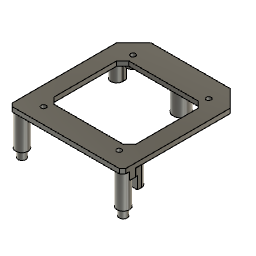
podstawka_bez_karoserii v3 (Autodesk Fusion 360 design; units mm, degrees)
Autodesk Fusion 360 part; units mm, degrees
note: some values were not read from the file. Set by a fixed rule: which face or edge a step refers to.
sketch "main" plane through (0, 0, 0) normal (0, 0, 1) x (1, 0, 0)
  circle A0 centre (50, 25) radius 4.065
  circle A1 centre (115.62, 25) radius 4.065
  circle A2 centre (50, 25) radius 2.6
  circle A3 centre (115.62, 25) radius 2.6
  line L0 (50, 29.065) -> (115.62, 29.065)
  line L1 (115.62, 29.065) -> (115.62, 90.235)
  line L2 (115.62, 90.235) -> (50, 90.235)
  line L3 (50, 90.235) -> (50, 27.6)
  line L4 (50, 29.065) -> (35.31, 29.065)
  line L5 (35.31, 29.065) -> (35.31, 90.235)
  line L6 (35.31, 90.235) -> (50, 90.235)
  line L7 (50, 90.235) -> (50, 29.065)
  line L8 (115.62, 29.065) -> (130.31, 29.065)
  line L9 (130.31, 29.065) -> (130.31, 90.235)
  line L10 (130.31, 90.235) -> (115.62, 90.235)
  line L11 (115.62, 90.235) -> (115.62, 29.065)
  line L12 (115.62, 59.65) -> (50, 59.65)
  line L13 (50, 59.65) -> (50, 90.235)
  line L14 (50, 90.235) -> (115.62, 90.235)
  line L15 (115.62, 90.235) -> (115.62, 59.65)
  line L16 (115.62, 59.65) -> (50, 90.235) construction
  line L17 (50, 59.65) -> (115.62, 90.235) construction
  line L18 (82.81, 74.9425) -> (82.81, 112.2058)
  circle A4 centre (82.81, 95.48) radius 5.245
  line L19 (82.81, 95.48) -> (88.055, 95.48)
  line L20 (82.81, 95.48) -> (77.565, 95.48)
  line L21 (77.565, 95.48) -> (77.565, 90.235)
  line L22 (88.055, 95.48) -> (88.055, 90.235)
  line L23 (50, 25) -> (54.065, 25)
  line L24 (50, 25) -> (45.935, 25)
  line L25 (54.065, 25) -> (54.065, 29.065)
  line L26 (45.935, 25) -> (45.935, 29.065)
  line L27 (115.62, 25) -> (115.62, 29.065)
  line L28 (115.62, 25) -> (119.685, 25)
  line L29 (119.685, 25) -> (119.685, 29.065)
  line L30 (111.555, 25) -> (111.555, 29.065)
  line L31 (115.62, 29.065) -> (100.93, 29.065)
  circle A5 centre (82.81, 95.48) radius 3
  line L32 (115.62, 90.235) -> (50, 29.065)
  circle A6 centre (115.62, 32.915) radius 3.85
  line L33 (115.62, 32.915) -> (119.47, 32.915)
  line L34 (115.62, 32.915) -> (111.77, 32.915)
  line L35 (119.47, 32.915) -> (119.47, 29.065)
  line L36 (111.77, 32.915) -> (111.77, 29.065)
  line L37 (115.62, 29.065) -> (50, 90.235)
  line L38 (53.85, 32.915) -> (53.85, 29.065)
  circle A7 centre (50, 32.915) radius 3.85
  line L39 (46.15, 32.915) -> (46.15, 29.065)
  line L40 (46.15, 86.385) -> (46.15, 90.235)
  circle A8 centre (50, 86.385) radius 3.85
  line L41 (53.85, 86.385) -> (53.85, 90.235)
  line L42 (111.77, 29.065) -> (119.47, 29.065)
  line L43 (119.47, 29.065) -> (119.47, 30.065)
  line L44 (119.47, 30.065) -> (111.77, 30.065)
  line L45 (111.77, 30.065) -> (111.77, 29.065)
  line L46 (46.15, 90.235) -> (53.85, 90.235)
  line L47 (53.85, 90.235) -> (53.85, 89.235)
  line L48 (53.85, 89.235) -> (46.15, 89.235)
  line L49 (46.15, 89.235) -> (46.15, 90.235)
  line L50 (50, 90.235) -> (82.81, 90.235)
  line L51 (82.81, 90.235) -> (82.81, 95.48)
  line L52 (82.81, 95.48) -> (50, 95.48)
  line L53 (50, 95.48) -> (50, 90.235)
  line L54 (130.31, 90.235) -> (82.81, 90.235)
  line L55 (82.81, 90.235) -> (82.81, 95.48)
  line L56 (50, 29.065) -> (115.62, 29.065)
  line L57 (115.62, 29.065) -> (115.62, 25)
  line L58 (115.62, 25) -> (50, 25)
  line L59 (50, 25) -> (50, 29.065)
  line L60 (45.935, 29.065) -> (119.685, 29.065)
  line L61 (119.685, 29.065) -> (119.685, 20.5)
  line L62 (119.685, 20.5) -> (45.935, 20.5)
  line L63 (45.935, 20.5) -> (45.935, 29.065)
  line L64 (88.055, 95.48) -> (115.62, 95.48)
  line L65 (115.62, 95.48) -> (115.62, 90.235)
  line L66 (115.62, 90.235) -> (88.055, 90.235)
  line L67 (88.055, 90.235) -> (88.055, 95.48)
  line L68 (50, 90.235) -> (115.62, 90.235)
  line L69 (115.62, 90.235) -> (115.62, 101.2915)
  line L70 (115.62, 101.2915) -> (50, 101.2915)
  line L71 (50, 101.2915) -> (50, 90.235)
  line L72 (46.15, 29.065) -> (46.15, 90.235)
  line L73 (119.685, 29.065) -> (119.685, 90.235)
  line L74 (119.685, 90.235) -> (115.62, 90.235)
  line L75 (115.62, 90.235) -> (115.62, 101.2915)
  line L76 (115.62, 101.2915) -> (119.685, 101.2915)
  line L77 (119.685, 101.2915) -> (119.685, 90.235)
  line L78 (46.15, 90.235) -> (50, 90.235)
  line L79 (50, 90.235) -> (50, 101.2915)
  line L80 (50, 101.2915) -> (46.15, 101.2915)
  line L81 (46.15, 101.2915) -> (46.15, 90.235)
  line L82 (82.81, 74.9425) -> (82.81, 57.8563)
  line L83 (46.15, 59.65) -> (115.62, 59.65)
  line L84 (90.31, 65.3563) -> (75.31, 65.3563)
  line L85 (75.31, 65.3563) -> (75.31, 50.3563)
  line L86 (75.31, 50.3563) -> (90.31, 50.3563)
  line L87 (90.31, 50.3563) -> (90.31, 65.3563)
  line L88 (90.31, 65.3563) -> (75.31, 50.3563) construction
  line L89 (75.31, 65.3563) -> (90.31, 50.3563) construction
  point P0 (82.81, 74.9425)
  point P1 (50, 59.65)
  point P2 (115.62, 59.65)
  point P3 (46.15, 59.65)
  point P4 (46.15, 59.65)
  point P5 (115.62, 59.65)
  point P6 (82.81, 74.9425)
  point P7 (82.81, 65.601)
  point P8 (82.81, 74.9425)
  point P9 (82.81, 57.8563)
  point P10 (82.81, 57.8563)
  dimension "d1" = 8.13
  dimension "d2" = 8.13
  dimension "d3" = 65.62
  dimension "d4" = 5.2
  dimension "d5" = 5.2
  dimension "d6" = 65.62
  dimension "d7" = 61.17
  dimension "d8" = 14.69
  dimension "d9" = 14.69
  dimension "d10" = 10.49
  dimension "d14" = 6
  dimension "d35" = 7.7
  dimension "d36" = 3.85
  dimension "d41" = 1
  dimension "d42" = 1
  dimension "d54" = 73.75
  dimension "d55" = 61.17
  dimension "d154" = 15
  dimension "d155" = 15
  constraint concentric A0 A2
  constraint concentric A1 A3
  constraint horizontal L0
  constraint vertical L1
  constraint horizontal L2
  constraint vertical L3
  constraint coincident A0 L0.start
  constraint coincident A2 L3.end
  constraint coincident L0.start L3
  constraint horizontal L4
  constraint vertical L5
  constraint horizontal L6
  constraint vertical L7
  constraint coincident L2.end L3.start
  constraint horizontal L8
  constraint vertical L9
  constraint horizontal L10
  constraint vertical L11
  constraint horizontal L12
  constraint perpendicular L12 L13
  constraint parallel L12 L14
  constraint parallel L13 L15
  constraint coincident L16 P8
  constraint coincident L17 P8
  constraint coincident L1.end L2.start
  constraint coincident P8 P6
  constraint vertical L18
  constraint coincident A4.centre L19.start
  constraint coincident A4 L19.end
  constraint perpendicular L18 L19
  constraint coincident A4 L20.end
  constraint perpendicular L18 L20
  constraint coincident L2 L21.end
  constraint tangent A4 L21
  constraint coincident L2 L22.end
  constraint tangent A4 L22
  constraint coincident A0.centre A2.centre
  constraint coincident A0 L23.end
  constraint perpendicular L3 L23
  constraint coincident A0 L24.end
  constraint parallel L23 L24
  constraint coincident L0 L25.end
  constraint tangent A0 L25
  constraint coincident L4 L26.end
  constraint tangent A0 L26
  constraint coincident A1.centre A3.centre
  constraint perpendicular L0 L27
  constraint coincident A1 L28.end
  constraint perpendicular L27 L28
  constraint coincident L8 L29.end
  constraint perpendicular L8 L29
  constraint symmetric L0.end L27 L1.start
  constraint symmetric L8.end L27 L31.end
  constraint symmetric L27 L28.end L30.start
  constraint symmetric L27 L29.end L30.end
  constraint coincident L0.end A6
  constraint coincident A6.centre L33.start
  constraint coincident A6 L33.end
  constraint perpendicular L1 L33
  constraint symmetric L1 A6.centre L33.start
  constraint symmetric L1 L33.end L34.end
  constraint coincident L8 L35.end
  constraint tangent A6 L35
  constraint symmetric L1 L35.end L36.end
  constraint symmetric L18 A6 A7
  constraint symmetric L18 L33.end L39.start
  constraint symmetric L18 L35.end L39.end
  constraint symmetric L18 L34.end L38.start
  constraint symmetric L18 L36.end L38.end
  constraint symmetric L12 L38.start L41.start
  constraint symmetric L12 L38.end L41.end
  constraint symmetric L12 A7 A8
  constraint symmetric L12 L39.start L40.start
  constraint symmetric L12 L39.end L40.end
  constraint horizontal L42
  constraint vertical L43
  constraint horizontal L44
  constraint vertical L45
  constraint horizontal L46
  constraint vertical L47
  constraint horizontal L48
  constraint vertical L49
  constraint horizontal L50
  constraint vertical L51
  constraint horizontal L52
  constraint vertical L53
  constraint horizontal L54
  constraint vertical L55
  constraint horizontal L56
  constraint vertical L57
  constraint horizontal L58
  constraint vertical L59
  constraint horizontal L60
  constraint vertical L61
  constraint horizontal L62
  constraint vertical L63
  constraint horizontal L64
  constraint vertical L65
  constraint horizontal L66
  constraint vertical L67
  constraint horizontal L68
  constraint vertical L69
  constraint horizontal L70
  constraint vertical L71
  constraint parallel L9 L73
  constraint horizontal L74
  constraint vertical L75
  constraint horizontal L76
  constraint vertical L77
  constraint horizontal L78
  constraint vertical L79
  constraint horizontal L80
  constraint vertical L81
  constraint coincident P1 L12.end
  constraint coincident P5 P2
  constraint midpoint L72 P4
  constraint coincident P10 P9
  constraint vertical L82
  constraint coincident P4 P3
  constraint horizontal L84
  constraint perpendicular L84 L85
  constraint parallel L84 L86
  constraint parallel L85 L87
  constraint coincident L88 P10
  constraint coincident L89 P10
  measures "d1" diameter of A0
  measures "d2" diameter of A1
  measures "d3" distance of A0.centre A1.centre
  measures "d4" diameter of A2
  measures "d5" diameter of A3
  measures "d6" distance of L0.start L0.end
  measures "d7" distance of L0.end L1.end
  measures "d8" distance of L0.start L4.end
  measures "d9" distance of L0.end L8.end
  measures "d10" diameter of A4
  measures "d14" diameter of A5
  measures "d35" diameter of A6
  measures "d36" distance of L2.end A8.centre
  measures "d41" distance of L36.end L44.end
  measures "d42" distance of L40.end L48.end
  measures "d54" distance of L26.end L29.end
  measures "d55" distance of L29.end L73.end
  measures "d154" distance of L85.end L86.end
  measures "d155" distance of L84.end L85.end
extrude "Extrude1" add sketch "main" along normal blind 3 contours A0 A2 L3 L23 L58 L59 | A0 A2 L23 L24 L58 | A0 L0 L25 L56 L60 | A0 A2 L3 L24 L59 | L0 L32 L38 A7 L56 L60 | L3 L7 A7 | A0 L4 L26 L60 L63 | L3 L7 L32 A7 | L4 A7 L39 L60 L72 | L32 A7 | A2 L23 L58 L59 | A2 L23 L24 L58 | L0 L31 L32 L36 L37 L38 L45 L56 L60 L85 L86 L87 | A1 L0 L30 L31 L42 L56 L60 | A1 A3 L28 L58 | A1 A3 L27 L57 L58 | A2 L24 L59 | L3 L7 A7 L72 L83 | L3 L7 L12 L32 L38 A7 L83 L85 | L4 L5 L6 L39 L40 L49 L60 L72 | L32 L38 A7 | A1 L8 L29 L42 L60 L61 | L1 L11 L37 L44 | L8 A6 L35 L42 L43 L44 L60 | A1 A3 L27 L28 L57 | L0 L31 A6 L36 L42 L44 L45 L56 L60 | L1 L11 A6 L44 | A6 L37 L44 | A3 L28 L58 | A3 L27 L57 L58 | L3 L7 L13 A8 L72 L83 | L3 L7 L12 L13 L37 A8 L41 L83 L84 L85 | L1 L11 A6 L34 L37 L44 | L1 L11 A6 L33 L44 | L1 L8 L10 L11 L15 A6 L35 L43 L54 L60 L73 L74 | A3 L27 L28 L57 | A6 L36 L37 L44 | A6 L37 L44 | A6 L35 L44 | L8 L9 L10 L54 L73 | L12 L32 L83 L85 | L32 L37 L85 L86 L87 | L3 L7 L13 A8 L48 | L3 L7 L13 L37 A8 L48 | L12 L37 L83 L84 L85 | L40 A8 L48 L72 | L1 L11 A6 L34 | L1 L11 A6 L33 | A6 L36 L37 | L12 L32 L83 L84 L87 | L32 L82 L84 | L12 L37 L83 L87 | L37 L82 L84 | L3 L7 L13 A8 L48 | L3 L7 L13 L37 L48 | L37 A8 L41 | L6 L40 A8 L46 L48 L49 L72 L78 | L1 L11 L12 A6 L36 L37 L83 L87 | L2 L14 L18 L32 L54 L66 L68 L82 L84 | L1 L11 L12 L15 L32 L83 L84 L87 | L2 L14 L18 L37 L41 L47 L50 L68 L82 L84 | L37 A8 L48 | L2 L14 A8 L41 L46 L47 L48 L50 L68 | L37 A8 L48 | L37 A8 L41 L48 | L2 L14 A4 L22 L54 L67 L68 | L18 A4 L20 A5 L51 L52 L55 | L2 L14 A4 L21 L50 L68 | L18 A4 L19 A5 L51 L55 | L18 A4 L19 A5 | L18 A4 L20 A5 L52 | L18 L20 A5 L51 L52 L55 | L18 L19 A5 L51 L55 | L18 L19 A5 | L18 L20 A5 L52 makes body 1
extrude "Extrude2" add sketch "main" against normal blind 18.7 contours L18 A4 L20 A5 L51 L52 L55 | L18 A4 L19 A5 L51 L55 | L18 A4 L19 A5 | L18 A4 L20 A5 L52 bodies 1
extrude "Extrude3" add sketch "main" against normal blind 5 contours L2 L14 A4 L22 L54 L67 L68 | L2 L14 A4 L21 L50 L68 | L18 L20 A5 L51 L52 L55 | L18 L19 A5 L51 L55 | L18 L19 A5 | L18 L20 A5 L52 bodies 1
extrude "Extrude4" add sketch "main" against normal blind 18.7 contours A2 L23 L58 L59 | A2 L23 L24 L58 | A2 L24 L59 | A3 L28 L58 | A3 L27 L57 L58 | A3 L27 L28 L57 bodies 1
extrude "Extrude5" add sketch "main" against normal blind 16.53 contours A0 A2 L3 L23 L58 L59 | A0 A2 L23 L24 L58 | A0 A2 L3 L24 L59 | A1 A3 L28 L58 | A1 A3 L27 L57 L58 | A1 A3 L27 L28 L57 bodies 1
extrude "Extrude6" add sketch "main" against normal blind 5 contours A0 L0 L25 L56 L60 | A0 L4 L26 L60 L63 | A1 L0 L30 L31 L42 L56 L60 | A1 L8 L29 L42 L60 L61 bodies 1
extrude "Extrude7" add 2 faces at (81.0617, 90.235, -1.6667) (86.3067, 90.235, -3.3333) along direction (0, -1, 0) blind 4 on bodies 1 bodies 1
extrude "Extrude8" add 4 faces at (51.355, 29.065, -1.6667) (48.645, 29.065, -1.6667) (116.975, 29.065, -1.6667) (112.91, 29.065, -1.6667) along direction (0, 1, 0) blind 4 on bodies 1 bodies 1
fillet "Fillet1" radius 5 2 faces at (114.265, 33.065, -1.6667) (48.645, 33.065, -1.6667) on bodies 1
fillet "Fillet2" radius 6 1 faces at (84.5583, 86.235, -3.3333) on bodies 1
move_face "OffsetFaces1" offset -3 1 faces at (130.31, 49.455, 1) on bodies 1
move_face "OffsetFaces2" offset -3 1 faces at (35.31, 49.455, 1) on bodies 1
extrude "Extrude9" cut sketch "main" against normal blind 18.7 contours L1 L11 L37 L44 | L8 A6 L35 L42 L43 L44 L60 | L0 L31 A6 L36 L42 L44 L45 L56 L60 | L1 L11 A6 L44 | A6 L37 L44 | L1 L11 A6 L34 L37 L44 | L1 L11 A6 L33 L44 | A6 L36 L37 L44 | A6 L37 L44 | A6 L35 L44 | L3 L7 L13 A8 L48 | L3 L7 L13 L37 A8 L48 | L40 A8 L48 L72 | L1 L11 A6 L34 | L1 L11 A6 L33 | L3 L7 L13 A8 L48 | L3 L7 L13 L37 L48 | L6 L40 A8 L46 L48 L49 L72 L78 | L37 A8 L48 | L2 L14 A8 L41 L46 L47 L48 L50 L68 | L37 A8 L48 | L37 A8 L41 L48 bodies 1
extrude "Extrude10" add sketch "main" against normal blind 18.7 separate body contours L1 L11 L37 L44 | L8 A6 L35 L42 L43 L44 L60 | L0 L31 A6 L36 L42 L44 L45 L56 L60 | L1 L11 A6 L44 | A6 L37 L44 | L1 L11 A6 L34 L37 L44 | L1 L11 A6 L33 L44 | A6 L36 L37 L44 | A6 L37 L44 | A6 L35 L44 | L3 L7 L13 A8 L48 | L3 L7 L13 L37 A8 L48 | L40 A8 L48 L72 | L1 L11 A6 L34 | L1 L11 A6 L33 | L3 L7 L13 A8 L48 | L3 L7 L13 L37 L48 | L6 L40 A8 L46 L48 L49 L72 L78 | L37 A8 L48 | L2 L14 A8 L41 L46 L47 L48 L50 L68 | L37 A8 L48 | L37 A8 L41 L48 makes body 2 at (111.7709, 32.8322, -12.4667) makes body 3 at (46.4381, 84.9238, -6.2333)
extrude "Extrude11" cut sketch "main" against normal blind 18.7 contours L3 L7 L13 A8 L48 | L3 L7 L13 L37 L48 | L6 L40 A8 L46 L48 L49 L72 L78 | L37 A8 L48 | L2 L14 A8 L41 L46 L47 L48 L50 L68 picked at (49.8114, 89.8877) picked at (51.28, 89.7227) bodies 3
extrude "Extrude12" add sketch "main" against normal blind 5 contours L3 L7 L13 A8 L48 | L3 L7 L13 L37 L48 | L6 L40 A8 L46 L48 L49 L72 L78 | L37 A8 L48 | L2 L14 A8 L41 L46 L47 L48 L50 L68 picked at (49.8114, 89.8877) picked at (51.28, 89.7227) bodies 1 3
extrude "Extrude13" cut sketch "main" against normal blind 18.7 contours L1 L11 L37 L44 | L8 A6 L35 L42 L43 L44 L60 | L0 L31 A6 L36 L42 L44 L45 L56 L60 | L1 L11 A6 L44 | A6 L37 L44 picked at (114.34, 29.5773) bodies 2
extrude "Extrude14" add sketch "main" against normal blind 5 contours L1 L11 L37 L44 | L8 A6 L35 L42 L43 L44 L60 | L0 L31 A6 L36 L42 L44 L45 L56 L60 | L1 L11 A6 L44 | A6 L37 L44 picked at (114.34, 29.5773) bodies 1 2
sketch "otwory" plane through (0, 0, 0) normal (0, 0, 1) x (1, 0, 0)
  circle A0 centre (58.31, 30.65) radius 3
  line L0 (115.62, 59.65) -> (50, 59.65)
  line L1 (82.81, 74.9425) -> (82.81, 112.2058)
  circle A1 centre (58.31, 88.65) radius 3
  circle A2 centre (107.31, 30.65) radius 3
  circle A3 centre (107.31, 88.65) radius 3
  line L2 (82.81, 74.9425) -> (82.81, 29)
  line L3 (54, 25) -> (82.81, 25)
  line L4 (82.81, 25) -> (82.81, 29)
  line L5 (82.81, 29) -> (54, 29)
  line L6 (54, 29) -> (54, 25)
  line L7 (111.555, 25) -> (82.81, 25)
  circle A4 through (61.31, 88.65, 3) (56.81, 91.2481, 3) (56.81, 86.0519, 3)
  circle A5 through (110.31, 88.65, 3) (105.81, 91.2481, 3) (105.81, 86.0519, 3)
  circle A6 through (110.31, 30.65, 3) (105.81, 33.2481, 3) (105.81, 28.0519, 3)
  circle A7 through (61.31, 30.65, 3) (56.81, 33.2481, 3) (56.81, 28.0519, 3)
  line L8 (59.8977, 27.9) -> (61.4854, 30.65)
  line L9 (61.4854, 30.65) -> (59.8977, 33.4)
  line L10 (59.8977, 33.4) -> (56.7223, 33.4)
  line L11 (56.7223, 33.4) -> (55.1346, 30.65)
  line L12 (55.1346, 30.65) -> (56.7223, 27.9)
  line L13 (56.7223, 27.9) -> (59.8977, 27.9)
  line L14 (105.7223, 27.9) -> (104.1346, 30.65)
  line L15 (104.1346, 30.65) -> (105.7223, 33.4)
  line L16 (105.7223, 33.4) -> (108.8977, 33.4)
  line L17 (108.8977, 33.4) -> (110.4854, 30.65)
  line L18 (110.4854, 30.65) -> (108.8977, 27.9)
  line L19 (108.8977, 27.9) -> (105.7223, 27.9)
  line L20 (55.1346, 88.65) -> (56.7223, 91.4)
  line L21 (56.7223, 91.4) -> (59.8977, 91.4)
  line L22 (59.8977, 91.4) -> (61.4854, 88.65)
  line L23 (61.4854, 88.65) -> (59.8977, 85.9)
  line L24 (59.8977, 85.9) -> (56.7223, 85.9)
  line L25 (56.7223, 85.9) -> (55.1346, 88.65)
  line L26 (104.1346, 88.65) -> (105.7223, 85.9)
  line L27 (105.7223, 91.4) -> (104.1346, 88.65)
  line L28 (108.8977, 91.4) -> (105.7223, 91.4)
  line L29 (110.4854, 88.65) -> (108.8977, 91.4)
  line L30 (108.8977, 85.9) -> (110.4854, 88.65)
  line L31 (105.7223, 85.9) -> (108.8977, 85.9)
  circle A8 centre (58.31, 30.65) radius 4
  circle A9 centre (107.31, 30.65) radius 4
  circle A10 centre (107.31, 88.65) radius 4
  circle A11 centre (58.31, 88.65) radius 4
  point P0 (111.555, 25)
  point P1 (58.31, 30.65)
  dimension "d51" = 6
  dimension "d52" = 29
  dimension "d53" = 24.5
  dimension "d68" = 6
  dimension "d69" = 2.75
  dimension "d70" = 5.5
  dimension "d71" = 6.3509
  dimension "d72" = 8
  dimension "d73" = 8
  dimension "d74" = 8
  dimension "d75" = 8
  constraint symmetric A0 L0 A1
  constraint symmetric A0 L1 A2
  constraint symmetric L1 A1 A3
  constraint coincident L1.start L2.start
  constraint perpendicular L0 L2
  constraint horizontal L3
  constraint vertical L4
  constraint horizontal L5
  constraint vertical L6
  constraint symmetric L3.end L4 L7.end
  constraint coincident P0 L7.start
  constraint coincident A0.centre A8.centre
  constraint symmetric L2 L8.start L14.start
  constraint symmetric L2 L8.end L14.end
  constraint symmetric L2 L9.end L15.end
  constraint symmetric L2 L10.end L16.end
  constraint symmetric L2 L11.end L17.end
  constraint symmetric L2 L12.end L18.end
  constraint symmetric L0 L8.start L21.end
  constraint symmetric L0 L8.end L22.end
  constraint symmetric L0 L9.end L23.end
  constraint symmetric L0 L10.end L24.end
  constraint symmetric L0 L11.end L20.start
  constraint symmetric L0 L12.end L20.end
  constraint symmetric L0 L14.start L27.start
  constraint symmetric L0 L14.end L26.start
  constraint symmetric L0 L15.end L26.end
  constraint symmetric L0 L16.end L30.start
  constraint symmetric L0 L17.end L29.start
  constraint symmetric L0 L18.end L28.start
  constraint coincident P1 A0.centre
  constraint concentric A2 A9
  constraint concentric A3 A10
  constraint concentric A1 A11
  measures "d51" diameter of A0
  measures "d52" distance of A0.centre L0
  measures "d53" distance of A0.centre L1
  measures "d69" distance of P1 L13
  measures "d70" distance of L10.end L12.end
  measures "d71" distance of L9.end L12.end
  measures "d72" diameter of A8
  measures "d73" diameter of A9
  measures "d74" diameter of A10
  measures "d75" diameter of A11
extrude "Extrude15" cut sketch "main" along normal blind 3 contours L4 L5 L6 L39 L40 L49 L60 L72 bodies 1
extrude "Extrude16" cut sketch "main" along normal blind 3 contours L8 L9 L10 L54 L73 bodies 1
extrude "Extrude17" add sketch "main" along normal blind 3 contours L10 L54 L65 L69 L74 L75 L76 L77 | L6 L46 L53 L71 L78 L79 L80 L81 | L2 L14 L22 L54 L64 L65 L66 L67 L68 L69 L75 | L2 L14 L21 L46 L50 L52 L53 L68 L71 L79 | L18 A4 L64 L69 L70 L75 | L18 A4 L52 L70 L71 L79 bodies 1
extrude "Extrude18" add sketch "main" along normal blind 3 contours A0 A1 L58 L61 L62 L63 | L0 L25 L30 L31 L56 L58 L60 bodies 1
hole "Hole1" at (107.31, 88.65, 0) at (58.31, 88.65, 0) at (58.31, 30.65, 0) at (107.31, 30.65, 0) direction (0, 0, 1) diameter 3.2 depth 3 tip angle 180 bodies 1
extrude "Extrude19" add sketch "otwory" against normal blind 2.4 contours A1 L22 | A1 L23 | A1 L21 | A1 L24 | A1 L20 | A1 L25 | A11 bodies 1
extrude "Extrude20" add sketch "otwory" against normal blind 2.4 contours A3 L29 | A3 L30 | A3 L28 | A3 L31 | A3 L27 | A3 L26 | A10 bodies 1
extrude "Extrude21" add sketch "otwory" against normal blind 2.4 contours A2 L17 | A2 L18 | A2 L16 | A2 L19 | A2 L15 | A2 L14 | A9 bodies 1
extrude "Extrude22" add sketch "otwory" against normal blind 2.4 contours A0 L9 | A0 L5 L8 L9 L10 L11 L12 A8 | A0 L5 L8 | A0 L5 L8 L12 L13 A8 | A0 L5 L8 | A0 L10 | A0 L5 L12 | A0 L5 L12 | A0 L13 | A0 L11 bodies 1
extrude "Extrude23" cut 1 faces at (53.5615, 24.798, -16.53) along direction (0, 0, 1) blind 0.2 on bodies 1 bodies 1
extrude "Extrude24" cut 1 faces at (117.6827, 27.9104, -16.53) along direction (0, 0, 1) blind 0.2 on bodies 1 bodies 1
extrude "Extrude25" add 1 faces at (50.3166, 26.3177, -18.7) along direction (0, 0, -1) blind 3.01 on bodies 1 bodies 1
extrude "Extrude26" add 1 faces at (115.8129, 25.8449, -18.7) along direction (0, 0, -1) blind 3.01 on bodies 1 bodies 1
extrude "Extrude27" add 1 faces at (115.5787, 34.2948, -18.7) along direction (0, 0, -1) blind 0.1 on bodies 1 bodies 1
extrude "Extrude28" add 1 faces at (48.7135, 87.425, -18.7) along direction (0, 0, -1) blind 0.1 on bodies 1 bodies 1
extrude "Extrude29" cut 1 faces at (78.344, 95.0704, -18.7) along direction (0, 0, 1) blind 3.87 on bodies 1 bodies 1
extrude "Extrude30" cut 1 faces at (51.2833, 89.235, -14.2) along direction (0, -1, 0) blind 0.3 on bodies 1 bodies 1
extrude "Extrude31" cut 1 faces at (114.3367, 30.065, -14.2) along direction (0, 1, 0) blind 0.3 on bodies 1 bodies 1
extrude "Extrude32" cut 1 faces at (48.7135, 87.325, -18.8) along direction (0, 0, 1) blind 10.8 on bodies 1 bodies 1
extrude "Extrude33" cut 1 faces at (115.5787, 34.2948, -18.8) along direction (0, 0, 1) blind 10.8 on bodies 1 bodies 1
extrude "Extrude34" add 2 faces at (115.8129, 25.8449, -21.71) (50.3166, 26.3177, -21.71) along direction (0, 0, -1) blind 5 on bodies 1 bodies 1
extrude "Extrude35" add 2 faces at (53.5615, 24.798, -16.33) (117.6827, 27.9104, -16.33) along direction (0, 0, -1) blind 5 on bodies 1 bodies 1
extrude "Extrude36" add 1 faces at (78.344, 95.0704, -14.83) along direction (0, 0, -1) blind 5 on bodies 1 bodies 1
extrude "Extrude37" add 2 faces at (115.5787, 34.2948, -8) (48.7135, 87.325, -8) along direction (0, 0, -1) blind 5 on bodies 1 bodies 1
extrude "Extrude38" cut 1 faces at (86.93, 91.1192, -5) along direction (0, 0, 1) blind 5 on bodies 1 bodies 1
extrude "Extrude39" cut 1 faces at (53.1931, 28.4493, -5) along direction (0, 0, 1) blind 5 on bodies 1 bodies 1
extrude "Extrude40" add 2 faces at (46.15, 72.2472, 2) (46.15, 88.085, -9.6667) along direction (-1, 0, 0) blind 0.215 on bodies 1 bodies 1
extrude "Extrude41" cut 1 faces at (84.5583, 90.0657, -3.3333) along direction (0, -1, 0) blind 10 on bodies 1 bodies 1
extrude "Extrude42" cut 1 faces at (48.645, 29.4047, -1.6667) along direction (0, 1, 0) blind 10 on bodies 1 bodies 1
extrude "Extrude43" cut 1 faces at (115.5187, 29.9279, -5) along direction (0, 0, 1) blind 5 on bodies 1 bodies 1
extrude "Extrude44" cut 1 faces at (111.6267, 29.4047, -3.3333) along direction (0, 1, 0) blind 10 on bodies 1 bodies 1
extrude "Extrude45" cut 1 faces at (119.5417, 29.4047, -3.3333) along direction (0, 1, 0) blind 10 on bodies 1 bodies 1
extrude "Extrude46" cut 1 faces at (114.3367, 30.365, -6) along direction (0, 1, 0) blind 10 on bodies 1 bodies 1
extrude "Extrude47" add sketch "main" against normal blind 13 contours L1 L11 A6 L34 L37 L44 | L1 L11 A6 L33 L44 | A6 L36 L37 L44 | A6 L37 L44 | A6 L35 L44 | L1 L11 A6 L34 | L1 L11 A6 L33 picked at (112.7238, 31.6234) bodies 1
extrude "Extrude48" add sketch "main" against normal blind 5 separate body contours L1 L11 L37 L44 | L8 A6 L35 L42 L43 L44 L60 | L0 L31 A6 L36 L42 L44 L45 L56 L60 | L1 L11 A6 L44 | A6 L37 L44 picked at (114.34, 29.5773) makes body 4
extrude "Extrude49" cut 1 faces at (45.935, 69.3922, 2) along direction (1, 0, 0) blind 0.215 on bodies 1 bodies 1
extrude "Extrude50" add sketch "main" against normal blind 5 contours A1 L0 L30 L31 L42 L56 L60 | A1 L8 L29 L42 L60 L61 bodies 1 4
extrude "Extrude51" cut 1 faces at (116.9033, 30.065, -10.3333) along direction (0, 1, 0) blind 0.3 on bodies 1 bodies 1
extrude "Extrude52" add sketch "main" against normal blind 5 contours A0 L0 L25 L56 L60 | A0 L4 L26 L60 L63 bodies 1
extrude "Extrude53" add sketch "main" against normal blind 5 contours L2 L14 A4 L22 L54 L67 L68 | L2 L14 A4 L21 L50 L68 bodies 1
extrude "Extrude54" add 1 faces at (50.0717, 29.065, -1.6667) along direction (0, 1, 0) blind 4 on bodies 1 bodies 1
extrude "Extrude55" add 2 faces at (81.0617, 90.235, -1.6667) (86.3067, 90.235, -3.3333) along direction (0, -1, 0) blind 5 on bodies 1 bodies 1
extrude "Extrude56" add 1 faces at (48.7167, 33.065, -3.3333) along direction (0, 1, 0) blind 1 on bodies 1 bodies 1
chamfer "Chamfer1" distance 5 angle 45 1 edges at (82.81, 85.235, -5) on bodies 1
chamfer "Chamfer2" distance 5 angle 45 1 edges at (50, 34.065, -5) on bodies 1
extrude "Extrude57" cut sketch "main" along normal blind 3 contours L12 L32 L83 L85 | L32 L37 L85 L86 L87 | L12 L37 L83 L84 L85 | L12 L32 L83 L84 L87 | L32 L82 L84 | L12 L37 L83 L87 | L37 L82 L84 bodies 1
extrude "Extrude58" cut 4 faces at (89.8505, 65.3563, 1) (86.891, 65.3563, 1) (80.7695, 65.3563, 1) (76.229, 65.3563, 1) along direction (0, 1, 0) blind 3.588 on bodies 1 bodies 1
extrude "Extrude59" cut 1 faces at (85.31, 68.9443, 1) along direction (0, 1, 0) blind 10 on bodies 1 bodies 1
extrude "Extrude60" cut 1 faces at (80.31, 50.3563, 1) along direction (0, -1, 0) blind 10 on bodies 1 bodies 1
extrude "Extrude61" cut 6 faces at (75.31, 57.3195, 1) (75.31, 51.8912, 1) (75.31, 47.023, 1) (75.31, 75.611, 1) (75.31, 66.5523, 1) (75.31, 63.4542, 1) along direction (-1, 0, 0) blind 10 on bodies 1 bodies 1
extrude "Extrude62" cut 6 faces at (90.31, 47.023, 1) (90.31, 51.1238, 1) (90.31, 54.9891, 1) (90.31, 61.5521, 1) (90.31, 66.5523, 1) (90.31, 75.611, 1) along direction (1, 0, 0) blind 10 on bodies 1 bodies 1
extrude "Extrude63" cut 1 faces at (100.31, 66.0817, 1) along direction (1, 0, 0) blind 5 on bodies 1 bodies 1
extrude "Extrude64" cut 1 faces at (65.31, 66.0817, 1) along direction (-1, 0, 0) blind 5 on bodies 1 bodies 1
extrude "Extrude65" cut 5 faces at (101.9767, 78.9443, 1) (93.6433, 78.9443, 1) (85.31, 78.9443, 1) (71.9767, 78.9443, 1) (63.6433, 78.9443, 1) along direction (0, 1, 0) blind 5 on bodies 1 bodies 1
extrude "Extrude66" cut 5 faces at (80.31, 40.3563, 1) (93.6433, 40.3563, 1) (101.9767, 40.3563, 1) (63.6433, 40.3563, 1) (71.9767, 40.3563, 1) along direction (0, -1, 0) blind 5 on bodies 1 bodies 1
extrude "Extrude67" cut 3 faces at (105.31, 38.6897, 1) (105.31, 66.0817, 1) (105.31, 82.2777, 1) along direction (1, 0, 0) blind 4 on bodies 1 bodies 1
extrude "Extrude68" cut 3 faces at (60.31, 82.2777, 1) (60.31, 66.0817, 1) (60.31, 38.6897, 1) along direction (-1, 0, 0) blind 4 on bodies 1 bodies 1
chamfer "Chamfer3" distance 4 angle 45 1 edges at (56.31, 35.3563, 1.5) on bodies 1
chamfer "Chamfer4" distance 4 angle 45 1 edges at (109.31, 35.3563, 1.5) on bodies 1
chamfer "Chamfer5" distance 4 angle 45 1 edges at (109.31, 83.9443, 1.5) on bodies 1
chamfer "Chamfer6" distance 4 angle 45 1 edges at (56.31, 83.9443, 1.5) on bodies 1
chamfer "Chamfer7" distance 11 angle 45 1 edges at (46.15, 101.2915, 1.5) on bodies 1
chamfer "Chamfer8" distance 11 angle 45 1 edges at (119.685, 101.2915, 1.5) on bodies 1
chamfer "Chamfer9" distance 2 angle 45 1 edges at (119.685, 20.5, 1.5) on bodies 1
chamfer "Chamfer10" distance 2 angle 45 1 edges at (46.15, 20.5, 1.5) on bodies 1
